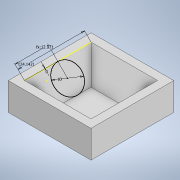
# Autodesk Inventor part: Part1
Saved by Autodesk Inventor 2021 (Build 250183000, 183)
## iProperties
Created: 2020-08-30
Part Number: Part1
Material: Generic
Document SubType Name: Modeling
Designer: deli
Density: 1 g/cm^3
Appearance: Default
Author: deli
Autodesk Inventor part; units mm, degrees
ref_plane "YZ Plane" through (0, 0, 0) normal (1, 0, 0) x (0, 1, 0)
ref_plane "XZ Plane" through (0, 0, 0) normal (0, 1, 0) x (-1, 0, 0)
ref_plane "XY Plane" through (0, 0, 0) normal (0, 0, 1) x (1, 0, 0)
sketch "Sketch1" plane through (0, 0, 0) normal (0, 1, 0) x (-1, 0, 0)
  line L0 (7.064, 6.8143) -> (-22.936, 6.8143)
  line L1 (-22.936, 6.8143) -> (-22.936, -23.1857)
  line L2 (-22.936, -23.1857) -> (7.064, -23.1857)
  line L3 (7.064, -23.1857) -> (7.064, 6.8143)
  point P0 (0, 0)
  dimension "d0" = 30
  dimension "d1" = 30
  constraints: 8 end point, 2 parallel, 1 horizontal, 1 perpendicular
  measures "d0" distance of L2.end L1.end
  measures "d1" distance of L1.end L0.end
extrude "Extrusion1" add sketch "Sketch1" along normal blind 10
sketch "Sketch2" plane through (0, 10, 0) normal (0, 1, 0) x (1, 0, 0)
  point P0 (0, 0)
sketch "Sketch3" plane through (0, 10, 0) normal (0, 1, 0) x (1, 0, 0)
  line L0 (2.936, 13.1857) -> (12.936, 13.1857)
  line L1 (12.936, 13.1857) -> (12.936, 3.1857)
  line L2 (12.936, 3.1857) -> (2.936, 3.1857)
  line L3 (2.936, 3.1857) -> (2.936, 13.1857)
  line L4 (22.936, -6.8143) -> (22.936, 23.1857) projected
  line L5 (-7.064, -6.8143) -> (22.936, -6.8143) projected
  point P0 (0, 0)
  dimension "d4" = 10
  dimension "d5" = 10
  dimension "d6" = 10
  dimension "d7" = 10
  constraints: 8 end point, 2 parallel, 1 horizontal, 1 perpendicular
  measures "d4" distance of L1.end L2.end
  measures "d5" distance of L0.end L1.end
  measures "d6" distance between parallel lines of L4 L1
  measures "d7" distance between parallel lines of L5 L2
extrude "Extrusion2" cut sketch "Sketch3" against normal blind 7.0711
chamfer "Chamfer1" distance 7.0711 distance2 7.0711 1 edges at (7.936, 10, -13.1857) measured on face at (6.2693, 10, -19.8524)
chamfer "Chamfer2" distance 7.0711 distance2 7.0711 1 edges at (2.936, 10, -8.1857) measured on face at (-3.7307, 10, -9.8524)
chamfer "Chamfer3" distance 7.0711 distance2 7.0711 1 edges at (7.936, 10, -3.1857) measured on face at (9.6026, 10, 3.481)
chamfer "Chamfer4" distance 7.0711 distance2 7.0711 1 edges at (12.936, 10, -8.1857) measured on face at (19.6026, 10, -9.8524)
sketch "Sketch4" plane through (-4.1351, 10, -20.2568) normal (0.7071, 0.7071, 0) x (-0.7071, 0.7071, 0)
  circle A0 centre (-5, 12.0711) radius 5
  line L0 (0, 0) -> (0, 24.1421) projected
  point P0 (-9.995, 20.2568)
  dimension "d22" = 10
  dimension "d23" = 0
  dimension "d24" = 24.1421
  dimension "d25" = 12.0711
  constraints: 1 centre point
  measures "d22" diameter of A0
  measures "d23" distance edge to line of A0 L0
  measures "d24" distance of L0.start L0.end
  measures "d25" vertical distance of A0.centre L0.end
equation "\"d7\" = d6"
equation "\"d25\" = 0.5 * d24"
body "Solid1"
